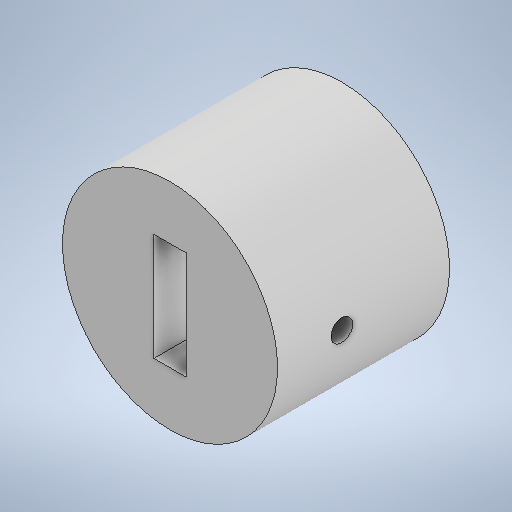
# Autodesk Inventor part: CS-Slider
Saved by Autodesk Inventor 2025.1 (Build 291241000, 241)
## iProperties
Created: 2025-04-02
Part Number: CS-Slider
Material: Generic
Document SubType Name: Modeling
Designer: a00584475
Density: 1 g/cm^3
Appearance: Default
Author: a00584475
Autodesk Inventor part; units mm, degrees
ref_plane "YZ Plane" through (0, 0, 0) normal (1, 0, 0) x (0, 1, 0)
ref_plane "XZ Plane" through (0, 0, 0) normal (0, 1, 0) x (-1, 0, 0)
ref_plane "XY Plane" through (0, 0, 0) normal (0, 0, 1) x (1, 0, 0)
sketch "Sketch1" plane through (0, 0, 0) normal (0, 0, 1) x (1, 0, 0)
  circle A0 centre (0, 0) radius 63.5
  dimension "d0" = 127
  constraints: 1 centre point, 1 coincident
  measures "d0" diameter of A0
extrude "Extrusion1" add sketch "Sketch1" against normal blind 101.6
sketch "Sketch2" plane through (0, 0, 0) normal (0, 0, 1) x (1, 0, 0)
  line L0 (-9.525, -31.75) -> (9.525, -31.75)
  line L1 (9.525, -31.75) -> (9.525, 31.75)
  line L2 (9.525, 31.75) -> (-9.525, 31.75)
  line L3 (-9.525, 31.75) -> (-9.525, -31.75)
  line L4 (-9.525, -31.75) -> (9.525, 31.75) construction
  line L5 (9.525, -31.75) -> (-9.525, 31.75) construction
  point P0 (0, 0)
  dimension "d3" = 63.5
  dimension "d4" = 19.05
  constraints: 12 end point, 2 midpoint, 2 parallel, 1 horizontal, 1 perpendicular
  measures "d3" distance of L0.end L1.end
  measures "d4" distance between parallel lines of L1 L3
extrude "Extrusion2" cut sketch "Sketch2" against normal blind 76.2
sketch "Sketch3" plane through (-9.525, -31.75, 0) normal (1, 0, 0) x (0, 0, -1)
  circle A0 centre (38.1, 31.75) radius 6.35
  line L0 (0, 0) -> (76.2, 0) projected
  line L1 (0, 0) -> (0, 63.5) projected
  point P0 (0, 31.75)
  dimension "d7" = 12.7
  dimension "d8" = 31.75
  dimension "d9" = 38.1
  constraints: 1 centre point
  measures "d7" diameter of A0
  measures "d8" distance from line of L0 A0.centre
  measures "d9" distance from line of L1 A0.centre
extrude "Extrusion3" cut sketch "Sketch3" along normal through all both and the other way through all
body "Solid1"
